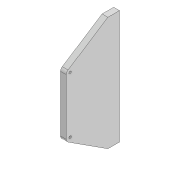
# Autodesk Inventor part: 202.001.05_Anbindung_Aktor
Saved by Autodesk Inventor 2021 (Build 250183000, 183)
## iProperties
Created: 2021-11-26
Part Number: 202.001.05_Anbindung_Aktor
Material: Generisch
Document SubType Name: Modeling
Designer: Oliver Ungerer
Density: 1 g/cm^3
Appearance: Vorgabe
Author: Oliver Ungerer
Autodesk Inventor part; units mm, degrees
ref_plane "YZ Plane" through (0, 0, 0) normal (1, 0, 0) x (0, 1, 0)
ref_plane "XZ Plane" through (0, 0, 0) normal (0, 1, 0) x (-1, 0, 0)
ref_plane "XY Plane" through (0, 0, 0) normal (0, 0, 1) x (1, 0, 0)
sketch "Skizze1" plane through (0, 0, 0) normal (1, 0, 0) x (0, 1, 0)
  line L0 (0, 0) -> (197, 0)
  line L1 (197, 0) -> (197, 92)
  line L2 (197, 92) -> (0, 92)
  line L3 (0, 92) -> (0, 0)
  dimension "d0" = 197
  dimension "d1" = 92
  constraints: 8 end point, 2 horizontal, 1 perpendicular, 1 vertical
  measures "d0" distance of L0.start L0.end
  measures "d1" distance of L0.end L1.end
extrude "Extrusion1" add sketch "Skizze1" along normal blind 10
sketch "Skizze2" plane through (10, 0, 0) normal (1, 0, 0) x (0, 0, -1)
  line L0 (-92, 0) -> (0, 0) projected
  line L1 (-85.5, 147) -> (-85.5, 50) construction
  line L2 (0, 0) -> (0, 197) projected
  dimension "d4" = 97
  dimension "d5" = 50
  dimension "d6" = 85.5
  constraints: 2 end point, 1 parallel
  measures "d4" distance of L1.end L1.start
  measures "d5" distance from line of L0 L1.end
  measures "d6" distance from line of L2 L1.start
hole "Bohrung1" at (10, 147, 85.5) at (10, 50, 85.5) direction (-1, 0, 0) diameter 4.2 depth 10 tip angle 118
sketch "Skizze3" plane through (10, 0, 0) normal (1, 0, 0) x (0, 0, -1)
  circle A0 centre (-85.5, 147) radius 2.1 projected
  circle A1 centre (-85.5, 50) radius 2.1 projected
  arc A2 (-92, 50) -> (-89.0242, 44.5383) centre (-85.5, 50) ccw
  arc A3 (-89.0242, 152.4617) -> (-92, 147) centre (-85.5, 147) ccw
  line L0 (0, 0) -> (0, 197) projected
  line L1 (0, 197) -> (-20, 197) construction
  line L2 (0, 0) -> (-20, 0) construction
  line L3 (-92, 0) -> (0, 0) projected
  line L4 (-20, 0) -> (-89.0242, 44.5383)
  line L5 (-20, 197) -> (-89.0242, 152.4617)
  line L6 (-92, 197) -> (-92, 0) projected
  line L7 (-20, 197) -> (-92, 197)
  line L8 (-92, 147) -> (-92, 197)
  line L9 (-92, 50) -> (-92, 0)
  line L10 (-92, 0) -> (-20, 0)
  dimension "d15" = 20
  constraints: 16 end point, 4 point on circle, 4 tangent, 3 point on line, 2 centre point, 2 coincident, 2 collinear, 1 horizontal, 1 perpendicular
  measures "d15" distance of L0.end L1.end
extrude "Extrusion2" cut sketch "Skizze3" against normal up to surface (10 mm away) contours A2 L4 L3 L6 | A3 L6 L7 L5
